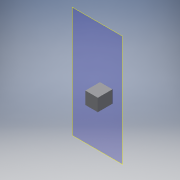
# Autodesk Inventor part: X motor
Saved by Autodesk Inventor 2016 (Build 200138000, 138)
## iProperties
Created: 2016-04-23
Part Number: X motor
Material: Generic
Document SubType Name: Modeling
Designer: Scott
Density: 1 g/cm^3
Appearance: Default
Author: Scott
Autodesk Inventor part; units mm, degrees
ref_plane "YZ Plane" through (0, 0, 0) normal (1, 0, 0) x (0, 1, 0)
ref_plane "XZ Plane" through (0, 0, 0) normal (0, 1, 0) x (-1, 0, 0)
ref_plane "XY Plane" through (0, 0, 0) normal (0, 0, 1) x (1, 0, 0)
ref_plane "Work Plane1" through (0.4503, 0, -6.096) normal (0, 0, -1) x (-1, 0, 0)
sketch "Sketch1" plane through (0.4503, 0, -6.096) normal (0, 0, -1) x (-1, 0, 0)
  line L0 (6.4269, 28.4846) -> (-36.7531, 28.4846)
  line L1 (-36.7531, 28.4846) -> (-36.7531, -14.6954)
  line L2 (-36.7531, -14.6954) -> (6.4269, -14.6954)
  line L3 (6.4269, -14.6954) -> (6.4269, 28.4846)
  line L4 (6.4269, 28.4846) -> (-36.7531, -14.6954) construction
  line L5 (-36.7531, 28.4846) -> (6.4269, -14.6954) construction
  point P0 (0.4503, 0)
  point P1 (-15.1631, 6.8946)
  dimension "d0" = 43.18
  dimension "d1" = 43.18
  constraints: 12 end point, 2 midpoint, 2 parallel, 1 horizontal, 1 perpendicular
  measures "d0" distance of L2.end L1.end
  measures "d1" distance of L1.end L0.end
extrude "Extrusion1" add sketch "Sketch1" against normal blind 50.8
body "Solid1"
